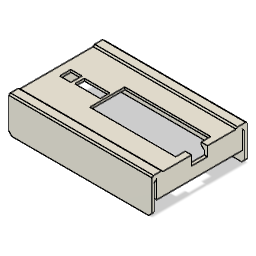
model (Autodesk Fusion 360 design; units mm, degrees)
Autodesk Fusion 360 part; units mm, degrees
sketch "Sketch1" plane through (0, 0, 0) normal (0, 1, 0) x (1, 0, 0)
  line L0 (41, -27) -> (-41, -27)
  line L1 (-41, -27) -> (-41, 27)
  line L2 (-41, 27) -> (41, 27)
  line L3 (41, 27) -> (41, -27)
  line L4 (41, -27) -> (-41, 27) construction
  line L5 (-41, -27) -> (41, 27) construction
  line L6 (-13, 11) -> (41, 11)
  line L7 (41, 11) -> (41, -11)
  line L8 (41, -11) -> (-13, -11)
  line L9 (-13, -11) -> (-13, 11)
  line L10 (-41, 3.5) -> (-32.5, 3.5)
  line L11 (-32.5, 3.5) -> (-32.5, -3.5)
  line L12 (-32.5, -3.5) -> (-41, -3.5)
  line L13 (-41, -3.5) -> (-41, 3.5)
  line L14 (-30.5, 3) -> (-14.5, 3)
  line L15 (-14.5, 3) -> (-14.5, -3)
  line L16 (-14.5, -3) -> (-30.5, -3)
  line L17 (-30.5, -3) -> (-30.5, 3)
  line L18 (45, 30) -> (-45, 30)
  line L19 (-45, 30) -> (-45, -30)
  line L20 (-45, -30) -> (45, -30)
  line L21 (45, -30) -> (45, 30)
  line L22 (45, 30) -> (-45, -30) construction
  line L23 (-45, 30) -> (45, -30) construction
  line L24 (41, 27) -> (45, 27)
  line L25 (45, 27) -> (45, 30)
  line L26 (45, 30) -> (41, 30)
  line L27 (41, 30) -> (41, 27)
  line L28 (41, -27) -> (45, -27)
  line L29 (45, -27) -> (45, -30)
  line L30 (45, -30) -> (41, -30)
  line L31 (41, -30) -> (41, -27)
  line L32 (-41, 27) -> (-45, 27)
  line L33 (-45, 27) -> (-45, 30)
  line L34 (-45, 30) -> (-41, 30)
  line L35 (-41, 30) -> (-41, 27)
  line L36 (-41, -27) -> (-45, -27)
  line L37 (-45, -27) -> (-45, -30)
  line L38 (-45, -30) -> (-41, -30)
  line L39 (-41, -30) -> (-41, -27)
  line L40 (43, 30) -> (43, -30)
  line L41 (-43, 30) -> (-43, -30)
  line L42 (-45, 28.5) -> (45, 28.5)
  line L43 (-45, -28.5) -> (45, -28.5)
  line L44 (-39.5, -3.5) -> (-37.7345, -3.5)
  line L45 (-37.7345, 3.5) -> (-39.5, 3.5)
  line L46 (-39.5, 3.5) -> (-39.5, -3.5)
  line L47 (-39.5, 3.5) -> (-32.5, 3.5)
  line L48 (-32.5, 0) -> (-30.5, 0)
  dimension "d1" = 82
  dimension "d2" = 54
  dimension "d3" = 90
  dimension "d4" = 60
  dimension "d22" = 54
  dimension "d23" = 22
  dimension "d24" = 8.5
  dimension "d25" = 7
  dimension "d26" = 16
  dimension "d49" = 6
  dimension "d50" = 2
  constraint horizontal L0
  constraint perpendicular L0 L1
  constraint parallel L0 L2
  constraint parallel L1 L3
  constraint coincident L4 origin
  constraint coincident L5 origin
  constraint horizontal L6
  constraint vertical L7
  constraint horizontal L8
  constraint vertical L9
  constraint horizontal L10
  constraint vertical L11
  constraint horizontal L12
  constraint vertical L13
  constraint horizontal L14
  constraint vertical L15
  constraint horizontal L16
  constraint vertical L17
  constraint horizontal L18
  constraint perpendicular L18 L19
  constraint parallel L18 L20
  constraint parallel L19 L21
  constraint coincident L22 origin
  constraint coincident L23 origin
  constraint horizontal L24
  constraint vertical L25
  constraint horizontal L26
  constraint vertical L27
  constraint horizontal L28
  constraint vertical L29
  constraint horizontal L30
  constraint vertical L31
  constraint horizontal L32
  constraint vertical L33
  constraint horizontal L34
  constraint vertical L35
  constraint horizontal L36
  constraint vertical L37
  constraint horizontal L38
  constraint vertical L39
  constraint midpoint L26 L40.start
  constraint midpoint L30 L40.end
  constraint midpoint L34 L41.start
  constraint midpoint L38 L41.end
  constraint midpoint L33 L42.start
  constraint midpoint L25 L42.end
  constraint midpoint L37 L43.start
  constraint midpoint L29 L43.end
  constraint midpoint L3 L7
  constraint midpoint L1 L13
  constraint horizontal L44
  constraint horizontal L45
  constraint vertical L46
  constraint coincident L10 L45.start
  constraint coincident L12 L44.start
  constraint perpendicular L11 L47
  constraint equal L11 L47
  constraint midpoint L11 L48.start
  constraint midpoint L17 L48.end
  constraint horizontal L48
  measures "d1" distance of L1.end L2.end
  measures "d2" distance of L0.end L1.end
  measures "d3" distance of L19.end L20.end
  measures "d4" distance of L18.end L19.end
  measures "d22" distance of L6.start L6.end
  measures "d23" distance of L6.start L8.end
  measures "d24" distance of L10.start L10.end
  measures "d25" distance of L10.end L11.end
  measures "d26" distance of L14.start L14.end
  measures "d49" distance of L14.end L15.end
  measures "d50" distance of L11 L17
extrude "Extrude1" add sketch "Sketch1" against normal blind 12 contours L21 L24 L28 L40 makes body 1
extrude "Extrude2" add sketch "Sketch1" 1 faces at (43.6667, 0, 9) along normal blind 1.5 contours L0 L31 L39 L43 | L0 L1 L2 L3 L6 L8 L9 L10 L11 L12 L44 L45 L47 | L3 L7 L24 L28 L40 | L28 L31 L40 L43 | L1 L13 L32 L36 L41 | L36 L39 L41 L43 | L21 L24 L28 L40 | L21 L28 L29 L40 L43 | L20 L30 L31 L40 L43 | L20 L31 L39 L43 | L1 L10 L12 L13 L46 | L19 L36 L37 L41 L43 | L19 L32 L36 L41 | L20 L38 L39 L41 L43 | L21 L24 L25 L40 L42 | L24 L27 L40 L42 | L20 L21 L29 L30 L40 L43 | L32 L35 L41 L42 | L19 L32 L33 L41 L42 | L19 L20 L37 L38 L41 L43 | L2 L27 L35 L42 | L18 L26 L27 L40 L42 | L18 L21 L25 L26 L40 L42 | L18 L19 L33 L34 L41 L42 | L18 L34 L35 L41 L42 | L18 L27 L35 L42 on bodies 1 bodies 1
extrude "Extrude3" add sketch "Sketch1" against normal blind 20 contours L20 L30 L31 L40 L43 | L20 L31 L39 L43 | L20 L38 L39 L41 L43 | L20 L21 L29 L30 L40 L43 | L19 L20 L37 L38 L41 L43 | L18 L26 L27 L40 L42 | L18 L21 L25 L26 L40 L42 | L18 L19 L33 L34 L41 L42 | L18 L34 L35 L41 L42 | L18 L27 L35 L42 bodies 1
sketch "Sketch2" plane through (45, 0, 0) normal (1, 0, 0) x (0, 0, -1)
  line L0 (-27, 0) -> (-27, -12)
  line L1 (-27, -12) -> (27, -12)
  line L2 (27, -12) -> (27, 0)
  line L3 (27, 0) -> (28.5, 0)
  line L4 (28.5, 0) -> (28.5, -20)
  line L5 (28.5, -20) -> (30, -20)
  line L6 (30, -20) -> (30, 1.5)
  line L7 (30, 1.5) -> (-30, 1.5)
  line L8 (-30, 1.5) -> (-30, -20)
  line L9 (-30, -20) -> (-28.5, -20)
  line L10 (-28.5, -20) -> (-28.5, 0)
  line L11 (-28.5, 0) -> (-27, 0)
  line L12 (5, 1.5) -> (-5, 1.5)
  line L13 (-5, 1.5) -> (-5, -4.5)
  line L14 (-5, -4.5) -> (5, -4.5)
  line L15 (5, -4.5) -> (5, 1.5)
  line L16 (5, 1.5) -> (-5, -4.5) construction
  line L17 (-5, 1.5) -> (5, -4.5) construction
  point P0 (0, -1.5)
  dimension "d29" = 10
  dimension "d30" = 6
  constraint horizontal L12
  constraint perpendicular L12 L13
  constraint parallel L12 L14
  constraint parallel L13 L15
  constraint coincident L16 P0
  constraint coincident L17 P0
  constraint midpoint L7 L12
  measures "d29" distance of L13.end L14.end
  measures "d30" distance of L12.start L14.end
extrude "Extrude5" add sketch "Sketch1" against normal blind 12 contours L19 L32 L36 L41 bodies 1
sketch "Sketch3" plane through (45, 0, 0) normal (1, 0, 0) x (0, 0, -1)
  line L0 (-27, 0) -> (-27, -12)
  line L1 (-27, -12) -> (27, -12)
  line L2 (27, -12) -> (27, 0)
  line L3 (27, 0) -> (28.5, 0)
  line L4 (28.5, 0) -> (28.5, -20)
  line L5 (28.5, -20) -> (30, -20)
  line L6 (30, -20) -> (30, 1.5)
  line L7 (30, 1.5) -> (-30, 1.5)
  line L8 (-30, 1.5) -> (-30, -20)
  line L9 (-30, -20) -> (-28.5, -20)
  line L10 (-28.5, -20) -> (-28.5, 0)
  line L11 (-28.5, 0) -> (-27, 0)
  line L12 (28.5, -14) -> (30.25, -14) construction
  line L13 (0, 0) -> (0, -13.7532)
  line L14 (28.5, -2) -> (26.5, 0)
  line L15 (-28.5, -2) -> (-26.5, 0)
  line L16 (28.5, -11) -> (26.5, -12)
  line L17 (26.5, -12) -> (28.5, -14)
  line L18 (-28.5, -11) -> (-26.5, -12)
  line L19 (-26.5, -12) -> (-28.5, -14)
  line L20 (30, 1.5) -> (29, 2.3)
  line L21 (29, 2.3) -> (24, 2.3)
  line L22 (24, 2.3) -> (23, 1.5)
  line L23 (-29, 2.3) -> (-24, 2.3)
  line L24 (-30, 1.5) -> (-29, 2.3)
  line L25 (-24, 2.3) -> (-23, 1.5)
  point P0 (-28.5, 0)
  point P1 (-27, -12)
  point P2 (-30, 1.5)
  point P3 (-30, 1.5)
  dimension "d31" = 11
  dimension "d32" = 2
  dimension "d33" = 2
  dimension "d38" = 1
  dimension "d40" = 2
  dimension "d41" = 2
  dimension "d52" = 1
  dimension "d53" = 5
  dimension "d54" = 1
  dimension "d55" = 0.8
  constraint horizontal L12
  constraint coincident L4 L12.start
  constraint coincident L13.start origin
  constraint coincident L4 L14.start
  constraint coincident L3 L14.end
  constraint symmetric L3.end L13 P0
  constraint symmetric L13 L14.start L15.start
  constraint symmetric L13 L14.end L15.end
  constraint coincident L4 L16.start
  constraint symmetric L1.end L13 P1
  constraint symmetric L12.start L13 L19.end
  constraint symmetric L16.start L13 L18.start
  constraint symmetric L13 L16.end L18.end
  constraint vertical L13
  constraint coincident L6.end L7.start
  constraint coincident L7 L22.end
  constraint horizontal L21
  constraint symmetric L6.end L13 P3
  constraint symmetric L13 L6.end P3
  constraint symmetric L13 L20.end L23.start
  constraint symmetric L13 L21.end L23.end
  constraint symmetric L13 L22.end L25.end
  measures "d31" distance of L3.end L16.start
  measures "d32" distance of L3.end L14.end
  measures "d33" distance of L3.end L14.start
  measures "d38" vertical distance of L16.start L16.end
  measures "d40" vertical distance of L12.start L16.end
  measures "d41" distance of L4 L16.end
  measures "d52" horizontal distance of L21.end L22.end
  measures "d53" distance of L20.end L21.end
  measures "d54" horizontal distance of L6.end L20.end
  measures "d55" vertical distance of L6.end L20.end
extrude "Extrude6" add sketch "Sketch3" against normal up to surface (90 mm away) contours L0 L10 L11 L15 | L7 L23 L24 L25 | L2 L3 L4 L14 | L7 L20 L21 L22 bodies 1
extrude "Extrude8" add sketch "Sketch3" against normal up to surface (90 mm away) separate body contours L0 L1 L18 | L0 L1 L10 L18 L19 | L1 L2 L16 | L1 L2 L4 L16 L17 makes body 2 at (15, -12, -28.5) makes body 3 at (15, -13, 28.5)
scale "Scale1" factors (0.9, 1, 1) about (0, 0, 0) bodies 2 3
combine "Combine1" operation add target body 1 tool bodies 2 3
sketch "Sketch4" plane through (0, 0, 27) normal (0, 0, 1) x (1, 0, 0)
  line L0 (-45, -0.5) -> (-45, -12)
  line L1 (-45, -12) -> (-43, -12)
  line L2 (-45, 0) -> (45, 0)
  line L3 (0, 0) -> (0, -12)
  line L4 (-43, -12) -> (-43, -0.5)
  line L5 (-43, 0) -> (-41, 0)
  line L6 (-43, 0) -> (-43, -2)
  line L7 (-43, -2) -> (-41, 0)
  line L8 (43, 0) -> (41, 0)
  line L9 (43, 0) -> (43, -2)
  line L10 (43, -2) -> (41, 0)
  line L11 (43, 0) -> (41, 0)
  line L12 (-43, -0.5) -> (-45, -0.5)
  point P0 (-43, 0)
  point P1 (43, -0.5)
  point P2 (43, 0)
  dimension "d47" = 2
  dimension "d48" = 2
  constraint coincident L3.start origin
  constraint perpendicular L2 L3
  constraint coincident P0 L5.start
  constraint perpendicular L4 L5
  constraint perpendicular L2 L6
  constraint symmetric L4.end L3 P1
  constraint symmetric P0 L3 P2
  constraint symmetric L3 P0 P2
  constraint symmetric L3 L5.end L8.end
  constraint symmetric L3 L6.end L9.end
  measures "d47" distance of P0 L5.end
  measures "d48" distance of P0 L6.end
extrude "Extrude7" add sketch "Sketch4" against normal up to surface (54 mm away) contours L2 L4 L5 L6 L7 | L2 L8 L9 L10 L11 bodies 1
extrude "Extrude4" cut sketch "Sketch2" against normal blind 10 contours L7 L12 L13 L14 L15 bodies 1
sketch "Sketch5" plane through (0, 0, 30) normal (0, 0, 1) x (1, 0, 0)
  line L0 (45, -20) -> (45, 1.5)
  line L1 (45, 1.5) -> (-45, 1.5)
  line L2 (-45, 1.5) -> (-45, -20)
  line L3 (-45, -20) -> (45, -20)
  line L4 (-43, -20) -> (-45, -18)
  line L5 (-43, -20) -> (-45, -20)
  line L6 (-45, -18) -> (-45, -20)
  line L7 (0, 0) -> (0, -20)
  line L8 (43, -20) -> (45, -18)
  line L9 (43, -20) -> (45, -20)
  line L10 (45, -18) -> (45, -20)
  point P0 (45, -20)
  dimension "d56" = 2
  constraint coincident L3 L4.start
  constraint coincident L2 L4.end
  constraint coincident L2.end L3.start
  constraint perpendicular L3 L6
  constraint equal L5 L6
  constraint coincident L7.start origin
  constraint midpoint L3 L7.end
  constraint symmetric L2.end L7 P0
  constraint symmetric L4.start L7 L8.start
  constraint symmetric L4.end L7 L8.end
  measures "d56" distance of L2.end L4.start
extrude "Extrude9" cut sketch "Sketch5" against normal up to surface (60 mm away) contours L0 L3 L8 L9 L10 | L2 L3 L4 L5 L6 bodies 1
